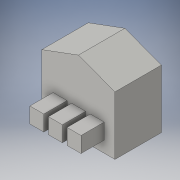
# Autodesk Inventor part: cwsumorobot
Saved by Autodesk Inventor 2016 (Build 200138000, 138)
## iProperties
Created: 2017-08-31
Part Number: cwsumorobot
Material: Generic
Document SubType Name: Modeling
Designer: student
Density: 1 g/cm^3
Appearance: Default
Author: student
Autodesk Inventor part; units mm, degrees
ref_plane "YZ Plane" through (0, 0, 0) normal (1, 0, 0) x (0, 1, 0)
ref_plane "XZ Plane" through (0, 0, 0) normal (0, 1, 0) x (-1, 0, 0)
ref_plane "XY Plane" through (0, 0, 0) normal (0, 0, 1) x (1, 0, 0)
sketch "Sketch1" plane through (0, 0, 0) normal (0, 0, 1) x (1, 0, 0)
  line L0 (-40, -4.6078) -> (40, -4.6078)
  line L1 (40, -4.6078) -> (40, 38.3746)
  line L2 (-40, 38.3746) -> (-40, -4.6078)
  line L3 (-40, 59.3419) -> (-40, 38.3746)
  line L4 (40, 59.3419) -> (40, 38.3746)
  line L5 (-40, 59.3419) -> (0, 74.1322)
  line L6 (0, 74.1322) -> (40, 59.3419)
  point P0 (0, 0)
  dimension "d0" = 80
  dimension "d5" = 78.74
  constraints: 14 end point, 1 horizontal, 1 parallel, 1 perpendicular, 1 vertical
  measures "d0" distance of L1.end L2.start
  measures "d5" vertical distance of L0.end L5.end
extrude "Extrusion1" add sketch "Sketch1" along normal blind 50.8
sketch "Sketch4" plane through (0, 0, 50.8) normal (0, 0, 1) x (1, 0, 0)
  line L0 (-27.6156, 7.8338) -> (-12.3756, 7.8338)
  line L1 (-12.3756, 7.8338) -> (-12.3756, 24.8882)
  line L2 (-12.3756, 24.8882) -> (-27.6156, 24.8882)
  line L3 (-27.6156, 24.8882) -> (-27.6156, 7.8338)
  line L4 (-7.2956, 7.8338) -> (7.9444, 7.8338)
  line L5 (7.9444, 7.8338) -> (7.9444, 24.8882)
  line L6 (7.9444, 24.8882) -> (-7.2956, 24.8882)
  line L7 (-7.2956, 24.8882) -> (-7.2956, 7.8338)
  line L8 (13.0244, 7.8338) -> (28.2644, 7.8338)
  line L9 (28.2644, 7.8338) -> (28.2644, 24.8882)
  line L10 (28.2644, 24.8882) -> (13.0244, 24.8882)
  line L11 (13.0244, 24.8882) -> (13.0244, 7.8338)
  point P0 (0, 0)
  dimension "d17" = 15.24
  dimension "d19" = 15.24
  dimension "d21" = 15.24
  constraints: 24 end point, 6 parallel, 3 horizontal, 3 perpendicular
  measures "d17" distance of L2.end L1.end
  measures "d19" distance of L6.end L5.end
  measures "d21" distance of L10.end L9.end
extrude "Extrusion2" add sketch "Sketch4" along normal blind 25.4
body "Solid1"
